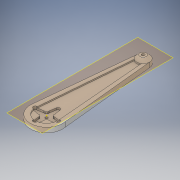
# Autodesk Inventor part: Delta_Arm
Saved by Autodesk Inventor 2019 (Build 230136000, 136)
## iProperties
Created: 2019-08-29
Part Number: Delta_Arm
Material: Generic
Document SubType Name: Modeling
Designer: Jorian Brusind
Density: 1 g/cm^3
Appearance: Default
Author: Jorian Brusind
Autodesk Inventor part; units mm, degrees
ref_plane "YZ Plane" through (0, 0, 0) normal (1, 0, 0) x (0, 1, 0)
ref_plane "XZ Plane" through (0, 0, 0) normal (0, 1, 0) x (-1, 0, 0)
ref_plane "XY Plane" through (0, 0, 0) normal (0, 0, 1) x (1, 0, 0)
sketch "Sketch1" plane through (0, 0, 0) normal (0, 1, 0) x (-1, 0, 0)
  circle A0 centre (0, 0) radius 25
  line L0 (0, 0) -> (0, -150)
  circle A1 centre (0, -150) radius 10
  line L1 (0, 0) -> (25, 0)
  line L2 (0, -150) -> (10, -150)
  line L3 (0, -150) -> (-10, -150)
  line L4 (0, 0) -> (-25, 0)
  line L5 (25, 0) -> (10, -150)
  line L6 (-25, 0) -> (-10, -150)
  dimension "d0" = 50
  dimension "d1" = 150
  dimension "d2" = 20
  constraints: 14 end point, 4 point on circle, 2 centre point, 2 coincident, 2 point on line, 1 horizontal, 1 parallel, 1 vertical
  measures "d0" diameter of A0
  measures "d1" distance of L0.start L0.end
  measures "d2" diameter of A1
extrude "Extrusion1" add sketch "Sketch1" along normal blind 7.5
sketch "Sketch2" plane through (0, 7.5, 0) normal (0, 1, 0) x (1, 0, 0)
  circle A0 centre (0, 0) radius 17.5
  arc A1 (10, 150) -> (-10, 150) centre (0, 150) ccw projected
  circle A2 centre (0, 150) radius 5
  line L0 (0, 0) -> (-17.5, 0)
  line L1 (0, 0) -> (17.5, 0)
  line L2 (0, 150) -> (-5, 150)
  line L3 (0, 150) -> (5, 150)
  line L4 (-17.5, 0) -> (-5, 150)
  line L5 (5, 150) -> (17.5, 0)
  dimension "d5" = 35
  dimension "d6" = 10
  constraints: 12 end point, 4 point on circle, 2 centre point, 2 coincident, 2 point on line, 1 horizontal, 1 parallel
  measures "d5" diameter of A0
  measures "d6" diameter of A2
extrude "Extrusion2" cut sketch "Sketch2" against normal blind 2 contours L4 A0 L5 L1 L0 | L4 A2 L5 A0
sketch "Sketch3" plane through (0, 5.5, 0) normal (0, 1, 0) x (1, 0, 0)
  arc A0 (5, 150) -> (-5, 150) centre (0, 150) ccw projected
  circle A1 centre (0, 150) radius 2.25
  circle A2 centre (0, 0) radius 2
  dimension "d9" = 4.5
  dimension "d12" = 4
  constraints: 2 centre point, 2 coincident
  measures "d9" diameter of A1
  measures "d12" diameter of A2
extrude "Extrusion4" cut sketch "Sketch3" against normal blind 5.5
sketch "Sketch4" plane through (0, 7.5, 0) normal (0, 1, 0) x (1, 0, 0)
  circle A0 centre (0, 150) radius 2.25 projected
  arc A1 (5, 150) -> (-5, 150) centre (0, 150) ccw projected
  arc A2 (10, 150) -> (-10, 150) centre (0, 150) ccw projected
  line L0 (24.505, 4.9505) -> (10, 150) projected
  circle A3 centre (0, 150) radius 10
  circle A4 centre (0, 150) radius 2.25
  point P0 (0, 0)
  dimension "d22" = 4.5
  constraints: 2 coincident, 1 centre point, 1 horizontal alignment, 2 other
  measures "d22" diameter of A4
ref_plane "Work Plane1" through (0, 12.5, 0) normal (0, 1, 0) x (1, 0, 0)
sketch "Sketch8" plane through (0, 5.5, 0) normal (0, 1, 0) x (1, 0, 0)
  point P0 (0, 0)
sketch "Sketch9" plane through (0, 7.5, 0) normal (0, 1, 0) x (1, 0, 0)
  arc A0 (2, 0) -> (-2, 0) centre (0, 0) ccw projected
  line L0 (17.5, 0) -> (-17.5, 0) projected
  circle A1 centre (0, 0) radius 17.5
  constraints: 1 coincident, 1 horizontal alignment, 2 other
extrude "Extrusion7" cut sketch "Sketch9" against normal blind 2 contours A0 L0 A1 | L0 A1
sketch "Sketch10" plane through (0, 7.5, 0) normal (0, 1, 0) x (1, 0, 0)
  arc A0 (-2.0881, -18.0545) -> (1.8643, -18.079) centre (-0.11, -17.7593) ccw
  line L0 (3.4056, -8.5599) -> (1.8643, -18.079)
  arc A1 (3.4056, -8.5599) -> (3.3448, -7.1465) centre (-0.0494, -8.0004) ccw
  arc A2 (4.0411, -5.092) -> (3.3448, -7.1465) centre (5.2844, -6.6585) ccw
  arc A3 (4.0411, -5.092) -> (5.0411, -4.1043) centre (0.0003, -0.0006) ccw
  arc A4 (7.1041, -3.4336) -> (5.0411, -4.1043) centre (6.5921, -5.367) ccw
  arc A5 (7.1041, -3.4336) -> (8.5166, -3.512) centre (8.0001, -0.0503) ccw
  line L1 (18.0541, -2.089) -> (8.5166, -3.512)
  arc A6 (18.0541, -2.089) -> (18.0787, 1.8634) centre (17.759, -0.1109) ccw
  line L2 (8.5596, 3.4047) -> (18.0787, 1.8634)
  arc A7 (8.5596, 3.4047) -> (7.1462, 3.344) centre (8.0001, -0.0503) ccw
  arc A8 (5.0917, 4.0402) -> (7.1462, 3.344) centre (6.6582, 5.2835) ccw
  arc A9 (5.0917, 4.0402) -> (4.104, 5.0402) centre (0.0003, -0.0006) ccw
  arc A10 (3.4333, 7.1032) -> (4.104, 5.0402) centre (5.3667, 6.5912) ccw
  arc A11 (3.4333, 7.1032) -> (3.5117, 8.5157) centre (0.05, 7.9993) ccw
  line L3 (2.0887, 18.0533) -> (3.5117, 8.5157)
  arc A12 (2.0887, 18.0533) -> (-1.8637, 18.0778) centre (0.1106, 17.7581) ccw
  line L4 (-3.405, 8.5587) -> (-1.8637, 18.0778)
  arc A13 (-3.405, 8.5587) -> (-3.3443, 7.1453) centre (0.05, 7.9993) ccw
  arc A14 (-4.0405, 5.0908) -> (-3.3443, 7.1453) centre (-5.2838, 6.6574) ccw
  arc A15 (-4.0405, 5.0908) -> (-5.0405, 4.1031) centre (0.0003, -0.0006) ccw
  arc A16 (-7.1035, 3.4325) -> (-5.0405, 4.1031) centre (-6.5915, 5.3658) ccw
  arc A17 (-7.1035, 3.4325) -> (-8.516, 3.5108) centre (-7.9996, 0.0491) ccw
  line L5 (-18.0536, 2.0878) -> (-8.516, 3.5108)
  arc A18 (-18.0536, 2.0878) -> (-18.0781, -1.8646) centre (-17.7585, 0.1097) ccw
  line L6 (-8.559, -3.4059) -> (-18.0781, -1.8646)
  arc A19 (-8.559, -3.4059) -> (-7.1456, -3.3451) centre (-7.9996, 0.0491) ccw
  arc A20 (-5.0911, -4.0414) -> (-7.1456, -3.3451) centre (-6.6577, -5.2847) ccw
  arc A21 (-5.0911, -4.0414) -> (-4.1034, -5.0414) centre (0.0003, -0.0006) ccw
  arc A22 (-3.4328, -7.1044) -> (-4.1034, -5.0414) centre (-5.3661, -6.5924) ccw
  arc A23 (-3.4328, -7.1044) -> (-3.5111, -8.5169) centre (-0.0494, -8.0004) ccw
  line L7 (-2.0881, -18.0545) -> (-3.5111, -8.5169)
  arc A24 (-18.2011, 3.0769) -> (-18.238, -2.8517) centre (-17.7585, 0.1097) ccw
  line L8 (-18.2011, 3.0769) -> (-8.6636, 4.4998)
  arc A25 (-6.8475, 4.3991) -> (-8.6636, 4.4998) centre (-7.9996, 0.0491) ccw
  arc A26 (-6.8475, 4.3991) -> (-5.816, 4.7345) centre (-6.5915, 5.3658) ccw
  arc A27 (-4.6622, 5.8741) -> (-5.816, 4.7345) centre (0.0003, -0.0006) ccw
  arc A28 (-4.6622, 5.8741) -> (-4.314, 6.9013) centre (-5.2838, 6.6574) ccw
  arc A29 (-4.3922, 8.7185) -> (-4.314, 6.9013) centre (0.05, 7.9993) ccw
  line L9 (-4.3922, 8.7185) -> (-2.8509, 18.2377)
  arc A30 (3.0777, 18.2008) -> (-2.8509, 18.2377) centre (0.1106, 17.7581) ccw
  line L10 (3.0777, 18.2008) -> (4.5007, 8.6633)
  arc A31 (4.4, 6.8472) -> (4.5007, 8.6633) centre (0.05, 7.9993) ccw
  arc A32 (4.4, 6.8472) -> (4.7353, 5.8157) centre (5.3667, 6.5912) ccw
  arc A33 (5.8749, 4.6619) -> (4.7353, 5.8157) centre (0.0003, -0.0006) ccw
  arc A34 (5.8749, 4.6619) -> (6.9022, 4.3137) centre (6.6582, 5.2835) ccw
  arc A35 (8.7194, 4.3919) -> (6.9022, 4.3137) centre (8.0001, -0.0503) ccw
  line L11 (8.7194, 4.3919) -> (18.2385, 2.8505)
  arc A36 (18.2017, -3.078) -> (18.2385, 2.8505) centre (17.759, -0.1109) ccw
  line L12 (18.2017, -3.078) -> (8.6642, -4.501)
  arc A37 (6.8481, -4.4003) -> (8.6642, -4.501) centre (8.0001, -0.0503) ccw
  arc A38 (6.8481, -4.4003) -> (5.8166, -4.7356) centre (6.5921, -5.367) ccw
  arc A39 (4.6627, -5.8753) -> (5.8166, -4.7356) centre (0.0003, -0.0006) ccw
  arc A40 (4.6627, -5.8753) -> (4.3146, -6.9025) centre (5.2844, -6.6585) ccw
  arc A41 (4.3927, -8.7197) -> (4.3146, -6.9025) centre (-0.0494, -8.0004) ccw
  line L13 (4.3927, -8.7197) -> (2.8514, -18.2388)
  arc A42 (-3.0772, -18.202) -> (2.8514, -18.2388) centre (-0.11, -17.7593) ccw
  line L14 (-3.0772, -18.202) -> (-4.5001, -8.6645)
  arc A43 (-4.3994, -6.8484) -> (-4.5001, -8.6645) centre (-0.0494, -8.0004) ccw
  arc A44 (-4.3994, -6.8484) -> (-4.7348, -5.8169) centre (-5.3661, -6.5924) ccw
  arc A45 (-5.8744, -4.663) -> (-4.7348, -5.8169) centre (0.0003, -0.0006) ccw
  arc A46 (-5.8744, -4.663) -> (-6.9016, -4.3149) centre (-6.6577, -5.2847) ccw
  arc A47 (-8.7188, -4.3931) -> (-6.9016, -4.3149) centre (-7.9996, 0.0491) ccw
  line L15 (-8.7188, -4.3931) -> (-18.238, -2.8517)
  point P0 (0, 0)
  point P1 (-0.0006, -0.0008)
  point P2 (5.0634, 6.1933)
  point P3 (0.0701, 8.4991)
  point P4 (0.0003, -0.0006)
  point P5 (11.2399, 13.7492)
  point P6 (5.0634, 6.1933)
  point P7 (6.1942, -5.0637)
  point P8 (13.7501, -11.2402)
  point P9 (-13.7495, 11.239)
  point P10 (-11.2393, -13.7504)
  point P11 (-5.0629, -6.1945)
  point P12 (-5.0629, -6.1945)
  point P13 (-0.0695, -8.5003)
  point P14 (0.0003, -0.0006)
  dimension "d38" = 0.001
  dimension "d39" = 1
  constraints: 96 point on circle, 48 centre point, 32 end point, 31 other
  measures "d38" distance of point (0, 0) point (-0.001, -0.001)
  measures "d39" distance between parallel lines of L6 L15
extrude "Extrusion8" cut sketch "Sketch10" against normal blind 5 contours L7 A23 A22 A21 A20 A19 L6 A18 L5 A17 A16 A15 A14 A13 L4 A12 L3 A11 A10 A9 A8 A7 L2 A6 L1 A5 A4 A3 A2 A1 L0 A0 | L8 A25 A26 A27 A28 A29 L9 A30 L10 A31 A32 A33 A34 A35 L11 A36 L12 A37 A38 A39 A40 A41 L13 A42 L14 A43 A44 A45 A46 A47 L15 A24
extrude "Extrusion9" add sketch "Sketch4" against normal blind 5
sketch "Sketch11" plane through (0, 7.5, 0) normal (0, 1, 0) x (1, 0, 0)
  circle A0 centre (0, 150) radius 2.25 projected
  line L0 (24.505, 4.9505) -> (10, 150) projected
  circle A1 centre (0, 150) radius 10
  point P0 (0, 0)
  constraints: 1 coincident, 1 horizontal alignment, 2 other
ref_plane "Work Plane2" through (0, 12.5, 0) normal (0, 1, 0) x (1, 0, 0)
sketch "Sketch12" plane through (0, 12.5, 0) normal (0, 1, 0) x (1, 0, 0)
  circle A0 centre (0, 150) radius 2.25 projected
  circle A1 centre (0, 150) radius 5
  point P0 (0, 0)
  dimension "d45" = 10
  constraints: 1 centre point, 1 coincident
  measures "d45" diameter of A1
loft "Loft3" add profiles "Sketch11", "Sketch12" contours A0 | A1 / A0 | A1
sketch "Sketch13" plane through (0, 12.5, -150) normal (0, 1, 0) x (1, 0, 0)
  circle A0 centre (0, 0) radius 2.25 projected
  circle A1 centre (0, 0) radius 2.25
  point P0 (0, -150)
  dimension "d50" = 4.5
  constraints: 1 centre point, 1 coincident
  measures "d50" diameter of A1
extrude "Extrusion10" cut sketch "Sketch13" against normal blind 10
body "Solid1"
